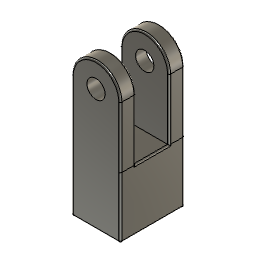
Mount for Quarter Twenty v5 (Autodesk Fusion 360 design; units mm, degrees)
Autodesk Fusion 360 part; units mm, degrees
sketch "Base" plane through (0, 0, 0) normal (0, 0, 1) x (1, 0, 0)
  circle A0 centre (0, 0) radius 6.425
  circle A1 centre (0, 0) radius 9.5
  dimension "d1" = 12.85
  dimension "d2" = 19
  constraint coincident A0.centre A1.centre
  measures "d1" diameter of A0
  measures "d2" diameter of A1
sketch "Sketch2" plane through (0, 0, 0) normal (0, 1, 0) x (1, 0, 0)
  line L0 (0, 0) -> (9.5, 0)
  line L1 (0, 0) -> (-9.5, 0)
  line L2 (-9.5, 0) -> (-9.5, -37.5)
  line L3 (-9.5, -37.5) -> (9.5, -37.5)
  line L4 (9.5, -37.5) -> (9.5, 0)
  dimension "d3" = 37.5
  constraint coincident L0.start L1.start
  constraint horizontal L0
  constraint parallel L0 L1
  constraint perpendicular L1 L2
  constraint perpendicular L2 L3
  constraint perpendicular L0 L4
  measures "d3" distance of L1.end L2.end
sketch "Sketch3" plane through (0, 0, 0) normal (0, 1, 0) x (1, 0, 0)
  circle A0 centre (0, -60) radius 1.5025
  arc A1 (-4, -60) -> (4, -60) centre (0, -60) ccw
  line L0 (-4, -60) -> (-4, -50)
  line L1 (-4, -50) -> (4, -50)
  line L2 (4, -50) -> (4, -60)
  dimension "d4" = 3.005
  dimension "d5" = 4
  constraint coincident A0.centre A1.centre
  constraint tangent A1 L0
  constraint vertical L0
  constraint perpendicular L0 L1
  constraint tangent A1 L2
  measures "d4" diameter of A0
  measures "d5" radius of A1
extrude "Extrude1" add sketch "Sketch3" along normal blind 2.5 from surface at 2.753 makes body 1
extrude "Extrude2" add sketch "Sketch3" against normal blind 2.5 from surface at -2.753 separate body makes body 2
sketch "Sketch4" plane through (0, 0, 0) normal (0, 1, 0) x (1, 0, 0)
  line L0 (-1.8054, -56.873) -> (-3.6107, -60)
  line L1 (-3.6107, -60) -> (-1.8054, -63.127)
  line L2 (-1.8054, -63.127) -> (1.8054, -63.127)
  line L3 (1.8054, -63.127) -> (3.6107, -60)
  line L4 (3.6107, -60) -> (1.8054, -56.873)
  line L5 (1.8054, -56.873) -> (-1.8054, -56.873)
  point P0 (0, -60)
  dimension "d12" = 3.127
  measures "d12" distance of P0 L5
extrude "Extrude3" cut sketch "Sketch4" along normal blind 0.753 from surface at 4.5 bodies 1
extrude "Extrude4" add 1 faces at (-1.3333, -3.5863, 50) along direction (0, 0, -1) blind 1 separate body on bodies 2 makes body 3
extrude "Extrude5" add 1 faces at (-1.3333, -5.253, 49.6667) along direction (0, 1, 0) blind 10.5 on bodies 3 bodies 3
extrude "Extrude10" add 1 faces at (1.3333, -1.753, 49) along direction (0, 0, -1) blind 9 on bodies 3 bodies 3
hole "Hole2" at (0, -0.003, 40) direction (0, 0, 1) diameter 5.118 depth 7.5 tip angle 180 bodies 3
thread "Thread2" "ANSI Unified Screw Threads 0.25 1/4-20 UNC 1B"
combine "Combine2" operation add target body 1 tool bodies 2 3
extrude "Extrude11" add 1 faces at (1.3333, 5.247, 43.3333) along direction (0, 1, 0) blind 0.006 on bodies 1 bodies 1
fillet "Fillet2" radius 0.25 20 edges at (-4, 2.753, 55) (0, 2.753, 64) (4, 2.753, 55) (-4, 0, 50) (4, 0, 50) (4, -2.753, 55) (0, -2.753, 64) (-4, -2.753, 55) (4, -5.253, 45) (4, -5.253, 55) (0, -5.253, 64) (-4, -5.253, 50) (-4, 5.253, 50) (0, 5.253, 64) (4, 5.253, 55) (4, 5.253, 45) (-4, 0, 40) (0, -5.253, 40) (0, 5.253, 40) (4, 0, 40) on bodies 1
thread "Thread3" "ANSI Unified Screw Threads 0.25 1/4-20 UNC 1B" major diameter 6.35 minor diameter 5.1181 pitch 1.27 angle 60 modelled right hand crest width 0.3461 on face at (0.2548, 2.5433, 42.5) crest through (-2.559, -0.003, 40.3175) on bodies 1
named bodies: "Quarter Twenty Camera Mount"
